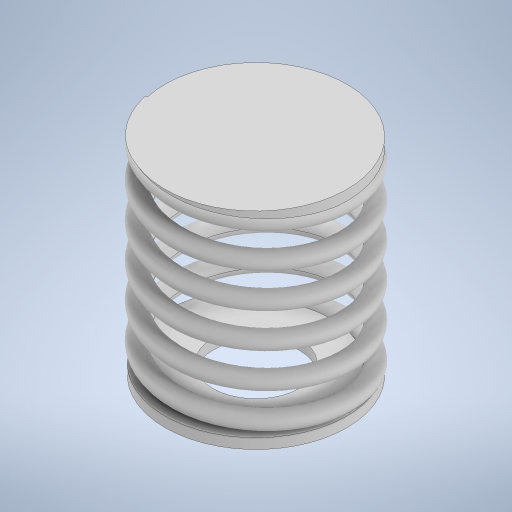
# Autodesk Inventor part: Spring
Saved by Autodesk Inventor 2024 (Build 280153000, 153)
## iProperties
Created: 2023-07-01
Part Number: Spring
Material: Generic
Document SubType Name: Modeling
Designer: vilas
Density: 1 g/cm^3
Appearance: Default
Author: vilas
Autodesk Inventor part; units mm, degrees
ref_plane "YZ Plane" through (0, 0, 0) normal (1, 0, 0) x (0, 1, 0)
ref_plane "XY Plane" through (0, 0, 0) normal (0, 0, 1) x (1, 0, 0)
sketch "Sketch1" plane through (0, 0, 0) normal (0, 0, 1) x (1, 0, 0)
  line L0 (0, 0) -> (-12.4, 0) construction
  circle A0 centre (-12.4, 0) radius 1.225
  dimension "d0" = 12.4
  dimension "d1" = 2.45
  constraints: 2 end point, 1 centre point, 1 coincident, 1 horizontal
  measures "d0" distance of L0.start L0.end
  measures "d1" diameter of A0
coil "Coil1" sketch "Sketch1" operation add axis through (0, -10, 0) along (0, 1, 0) pitch 5.08 turns 5.965 hand left
ref_plane "Work Plane1" through (0, 30.3, 0) normal (0, 1, 0) x (-1, 0, 0)
sketch "Sketch2" plane through (0, 30.3, 0) normal (0, 1, 0) x (-1, 0, 0)
  circle A0 centre (0, 0) radius 13.35
  dimension "d11" = 26.7
  constraints: 1 centre point, 1 coincident
  measures "d11" diameter of A0
extrude "Extrusion1" add sketch "Sketch2" against normal blind 1.5
sketch "Sketch3" plane through (0, 0, 0) normal (0, 1, 0) x (-1, 0, 0)
  circle A0 centre (0, 0) radius 13.35
  circle A1 centre (0, 0) radius 6.35
  dimension "d14" = 26.7
  dimension "d15" = 12.7
  constraints: 2 centre point, 2 coincident
  measures "d14" diameter of A0
  measures "d15" diameter of A1
extrude "Extrusion2" add sketch "Sketch3" along normal blind 1.5
sketch "Sketch4" plane through (0, 0, 0) normal (1, 0, 0) x (0, 1, 0)
  line L0 (0, -13.35) -> (0, 13.35) projected
  line L1 (0, 13.35) -> (-1.5, 13.35)
  line L2 (-1.5, 13.35) -> (-1.5, -13.35)
  line L3 (-1.5, -13.35) -> (0, -13.35)
  line L4 (0, -13.35) -> (0, 13.35)
  line L5 (30.3, -13.35) -> (30.3, 13.35) projected
  line L6 (30.3, 13.35) -> (31.8, 13.35)
  line L7 (31.8, 13.35) -> (31.8, -13.35)
  line L8 (31.8, -13.35) -> (30.3, -13.35)
  line L9 (30.3, -13.35) -> (30.3, 13.35)
  point P0 (0, 0)
  point P1 (0, -10.9098)
  point P2 (30.3, 12.3394)
  point P3 (30.3, 2.9122)
  dimension "d18" = 1.5
  dimension "d19" = 26.7
  dimension "d20" = 1.5
  dimension "d21" = 26.7
  constraints: 16 end point, 4 parallel, 2 horizontal, 2 perpendicular
  measures "d18" distance of L3.end L2.end
  measures "d19" distance of L2.end L1.end
  measures "d20" distance of L7.end L8.end
  measures "d21" distance of L6.end L7.end
extrude "Extrusion3" cut sketch "Sketch4" along normal through all both and the other way through all
body "Solid1"
